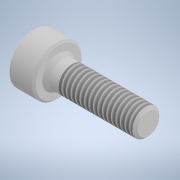
# Autodesk Inventor part: ISO-4762 M3x10
Saved by Autodesk Inventor 2021 (Build 250183000, 183)
## iProperties
Created: 2026-04-25
Part Number: ISO-4762 M3x10
Material: Generic
Catalog Web Link: www.3dfindit.com
Description: ISO-4762-Cylinder head screws cap screws
Vendor: FESTO
Document SubType Name: Modeling
Designer: psAdmin
Manufacturer: FESTO
Mass: 0.132895 g
Surface Area: 1.96088 cm^2
Volume: 0.132895 cm^3
Density: 1 g/cm^3
Appearance: PSOLRGB-176-176-176
Category: PARTsolutions
Company: FESTO
Title: ISO-4762 M3x10
Author: Cadenas PARTsolutions
Comments: Cylinder head screws cap screws
PSOL_IDENT_0: {$CADENAS_DATA/23d-libs/festo/zyl_zubeh/din_4762/din_en_iso_4762.prj},171 {VTYP=3D},{NB=ISO-4762 M3x
PSOL_IDENT_1: 10},{LINA=ISO-4762 M3x10},{NN=ISO-4762},{DATE=17.04.2026 14:13:08},{GEOMDATE=10.04.2026 13:28:17},{V
PSOL_IDENT_2: ERSION=},{LINEID=310},{WBVAR=},{WBNUMERIC=}  {NB=ISO-4762 M3x10},{LINA=ISO-4762 M3x10},{KT=DUMMY},{I
PSOL_IDENT_3: DNR=},{D=3.000},{D3=2.387},{P=0.500},{L=10.000},{B=8.5},{BX=18.000},{LS=0},{LG=1.5},{DK=5.500},{DA=3
PSOL_IDENT_4: .600},{DS=3.000},{E=2.870},{LF=0.510},{K=3.000},{R=0.100},{S=2.500},{T=1.300},{V=0.300},{DW=5.070},{
PSOL_IDENT_5: W=1.150},{NENN=M3x10}
NB: ISO-4762 M3x10
NN: ISO-4762
NT: Cylinder head screws cap screws
NBSYN: ISO-4762 $NENN.
LINA: ISO-4762 M3x10
CATALOG: Festo
ROWDESC: M3x10
D: 3
D3: 2.387
P: 0.5
L: 10
B: 8.5
LS: 0
LG: 1.5
DK: 5.5
DA: 3.6
DS: 3
E: 2.87
LF: 0.51
K: 3
R: 0.1
S: 2.5
T: 1.3
V: 0.3
DW: 5.07
W: 1.15
SUPPLIER: FESTO
ARTICLENO: ISO-4762 M3x10
BOMINFO: ISO-4762 M3x10
CREATOR: CADENAS GmbH
Autodesk Inventor part; units mm, degrees
sketch "Sketch_1" plane through (0, 0, 0) normal (0, 0, 1) x (1, 0, 0)
  line L0 (10, 0) -> (-3, 0)
  line L1 (-3, 0) -> (-3, 2.75)
  line L2 (-3, 2.75) -> (0, 2.75)
  line L3 (0, 2.75) -> (0, 1.8)
  line L4 (0, 1.8) -> (0.51, 1.5)
  line L5 (0.51, 1.5) -> (9.6935, 1.5)
  line L6 (9.6935, 1.5) -> (10, 1.1935)
  line L7 (10, 1.1935) -> (10, 0)
  line L8 (10, 0) -> (-3, 0)
  constraints: 18 end point
revolve "Revolution1" add sketch "Sketch_1" angle 360 about axis through (10, 0, 0) along (1, 0, 0)
thread "Thread1" size "M3x0.5" class "6g" standard "ISO Metric profile" length 8.1935
sketch "Sketch_6" plane through (0, 0, 0) normal (0, 0, 1) x (1, 0, 0)
  line L0 (0, 0) -> (-3, 0)
  line L1 (-3, 3.3) -> (-3, 2.45)
  line L2 (-3, 2.45) -> (-2.7, 2.75)
  line L3 (-2.7, 2.75) -> (-0.215, 2.75)
  line L4 (-0.215, 2.75) -> (0, 2.535)
  line L5 (0, 2.535) -> (0, 3.3)
  line L6 (0, 3.3) -> (-3, 3.3)
  constraints: 14 end point
revolve "Revolution2" cut sketch "Sketch_6" angle 360 about axis through (0, 0, 0) along (1, 0, 0)
sketch "Sketch3" plane through (-3, 0, 0) normal (-1, 0, 0) x (0, 0, 1)
  point P0 (0, 0)
hole "Hole1" at (-3, 0, 0) direction (1, 0, 0) diameter 2.5 depth 1.3 tip angle 120 countersink diameter 2.85 countersink angle 90
sketch "Sketch_2" plane through (-3, 0, 0) normal (1, 0, 0) x (0, 0, -1)
  line L0 (-1.25, -0.7217) -> (0, -1.4434)
  line L1 (0, -1.4434) -> (1.25, -0.7217)
  line L2 (1.25, -0.7217) -> (1.25, 0.7217)
  line L3 (1.25, 0.7217) -> (0, 1.4434)
  line L4 (0, 1.4434) -> (-1.25, 0.7217)
  line L5 (-1.25, 0.7217) -> (-1.25, -0.7217)
  constraints: 12 end point
extrude "Extrusion1" cut sketch "Sketch_2" along normal mid plane 2.6
ref_plane "ANBAU_XY" through (0, 0, 0) normal (-1, 0, 0) x (0, 0, -1)
ref_plane "ANBAU_YZ" through (0, 0, 0) normal (0, 0, -1) x (0, -1, 0)
ref_plane "ANBAU_ZX" through (0, 0, 0) normal (0, -1, 0) x (-1, 0, 0)
ref_plane "IP1_XY" through (0, 0, 0) normal (1, 0, 0) x (0, 0, -1)
ref_plane "IP1_YZ" through (0, 0, 0) normal (0, 0, -1) x (0, 1, 0)
ref_plane "IP1_ZX" through (0, 0, 0) normal (0, 1, 0) x (1, 0, 0)
ref_plane "IP2_XY" through (-3, 0, 0) normal (1, 0, 0) x (0, 0, -1)
ref_plane "IP2_YZ" through (-3, 0, 0) normal (0, 0, -1) x (0, 1, 0)
ref_plane "IP2_ZX" through (-3, 0, 0) normal (0, 1, 0) x (1, 0, 0)
ref_plane "IP3_XY" through (10, 0, 0) normal (1, 0, 0) x (0, 0, -1)
ref_plane "IP3_YZ" through (10, 0, 0) normal (0, 0, -1) x (0, 1, 0)
ref_plane "IP3_ZX" through (10, 0, 0) normal (0, 1, 0) x (1, 0, 0)
body "Solid1"
